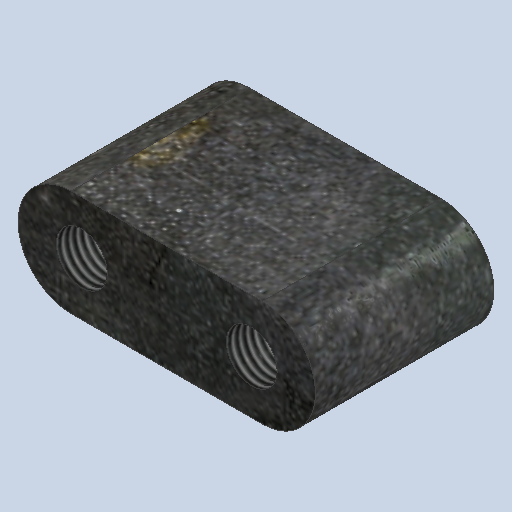
# Autodesk Inventor part: Topo Macaco
Saved by Autodesk Inventor 2024 (Build 280153000, 153)
## iProperties
Created: 2024-06-03
Part Number: Topo Macaco
Material: Steel ASTM A36
Document SubType Name: Modeling
Designer: Pedro
Density: 7.85 g/cm^3
Appearance: Plate
Mass: 458.177 g
Surface Area: 130.248 cm^2
Volume: 58.3665 cm^3
Author: Pedro
Autodesk Inventor part; units mm, degrees
ref_plane "YZ Plane" through (0, 0, 0) normal (1, 0, 0) x (0, 1, 0)
ref_plane "XZ Plane" through (0, 0, 0) normal (0, 1, 0) x (-1, 0, 0)
ref_plane "XY Plane" through (0, 0, 0) normal (0, 0, 1) x (1, 0, 0)
sketch "Sketch1" plane through (0, 0, 0) normal (0, 0, 1) x (1, 0, 0)
  line L0 (-35, 12.5) -> (35, 12.5)
  line L1 (35, 12.5) -> (35, -12.5)
  line L2 (35, -12.5) -> (-35, -12.5)
  line L3 (-35, -12.5) -> (-35, 12.5)
  point P0 (0, 0)
  dimension "d0" = 70
  dimension "d1" = 25
  dimension "d2" = 35
  dimension "d3" = 12.5
  constraints: 8 end point, 2 parallel, 1 horizontal, 1 perpendicular
  measures "d0" distance of L0.start L0.end
  measures "d1" distance of L0.end L1.end
  measures "d2" distance from line of L3 point (0, 0)
  measures "d3" distance from line of L2 point (0, 0)
extrude "Extrusion1" add sketch "Sketch1" along normal blind 42
full round fillet "Full Round Fillet1" first side at (11.6667, 12.5, 14) centre faces at (-35, 4.1667, 14) second side at (-11.6667, -12.5, 14)
full round fillet "Full Round Fillet2" first side at (15.8333, 12.5, 14) centre faces at (35, -4.1667, 14) second side at (-3.3334, -12.5, 28)
sketch "Sketch2" plane through (0, 0, 42) normal (0, 0, 1) x (1, 0, 0)
  circle A0 centre (-20, 0) radius 6
  circle A1 centre (20, 0) radius 6
  point P0 (0, 0)
  dimension "d6" = 12
  dimension "d7" = 12
  dimension "d8" = 40
  dimension "d9" = 20
  constraints: 2 centre point
  measures "d6" diameter of A0
  measures "d7" diameter of A1
  measures "d8" distance of A0.centre A1.centre
  measures "d9" distance of point (0, 0) A0.centre
extrude "Extrusion2" cut sketch "Sketch2" against normal blind 42
thread "Thread1" size "M12x1.75" class "6H" standard "ANSI Metric M Profile" full length
thread "Thread2" size "M12x1.75" class "6H" standard "ANSI Metric M Profile" full length
body "Solid1"
